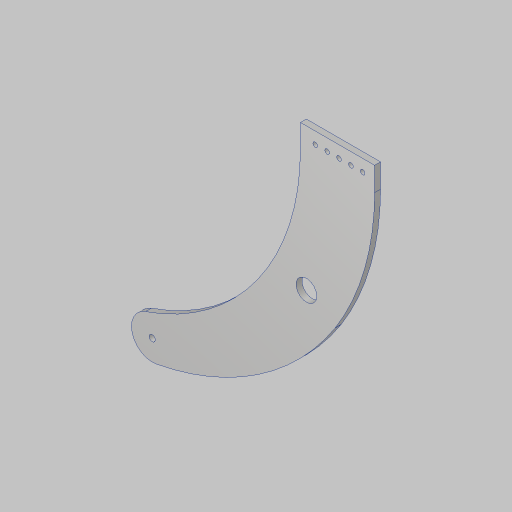
# Autodesk Inventor part: CL7-008
Saved by Autodesk Inventor 2023.5 (Build 275446000, 446)
## iProperties
Created: 2025-03-17
Part Number: CL7-008
Material: Aluminum 6061
Document SubType Name: Modeling
Designer: slick
Density: 2.7 g/cm^3
Appearance: Aluminum - Flat
Author: slick
Autodesk Inventor part; units mm, degrees
ref_plane "YZ Plane" through (0, 0, 0) normal (1, 0, 0) x (0, 1, 0)
ref_plane "XZ Plane" through (0, 0, 0) normal (0, 1, 0) x (-1, 0, 0)
ref_plane "XY Plane" through (0, 0, 0) normal (0, 0, 1) x (1, 0, 0)
sketch "Sketch1" plane through (0, 0, 0) normal (0, 0, 1) x (1, 0, 0)
  line L0 (-149.225, 152.4) -> (73.025, 152.4) construction
  line L1 (73.025, 152.4) -> (73.025, 127) construction
  line L2 (73.025, 127) -> (-149.225, 127) construction
  line L3 (-149.225, 127) -> (-149.225, 152.4) construction
  circle A0 centre (-165.1, -127) radius 12.7 construction
  circle A1 centre (0, 0) radius 23.8125 construction
  circle A2 centre (0, 0) radius 11.1125
  circle A3 centre (0, 0) radius 36.5125 construction
  line L4 (73.025, 152.4) -> (73.025, 127)
  line L5 (73.025, 152.4) -> (-6.4223, 152.4)
  line L6 (-6.4223, 152.4) -> (-6.4223, 127)
  circle A4 centre (-165.1, -127) radius 22.225 construction
  arc A5 (-172.3658, -105.9962) -> (-6.4223, 127) centre (-252.9655, 127) ccw
  arc A6 (-160.9917, -148.842) -> (30.7123, -19.7463) centre (-214.9861, 138.2242) ccw
  arc A7 (-172.3658, -105.9962) -> (-160.9917, -148.842) centre (-165.1, -127) ccw
  arc A8 (30.9373, -19.3918) -> (73.025, 127) centre (-202.6133, 127) ccw
  arc A9 (30.7123, -19.7463) -> (30.9373, -19.3918) centre (0, 0) ccw
  point P0 (60.325, 139.7)
  point P1 (73.025, 139.7)
  point P2 (47.625, 139.7)
  point P3 (34.925, 139.7)
  point P4 (22.225, 139.7)
  point P5 (9.525, 139.7)
  point P6 (30.9373, -19.3918)
  dimension "d0" = 25.4
  dimension "d1" = 127
  dimension "d2" = 222.25
  dimension "d3" = 149.225
  dimension "d4" = 25.4
  dimension "d5" = 127
  dimension "d6" = 165.1
  dimension "d7" = 12.7
  dimension "d8" = 47.625
  dimension "d9" = 22.225
  dimension "d12" = 12.7
  dimension "d17" = 12.7
  dimension "d18" = 9.525
  dimension "d19" = 292.1
  constraints: 15 point on circle, 14 end point, 10 centre point, 7 tangent, 5 coincident, 2 horizontal, 2 parallel, 2 perpendicular, 2 point on line, 1 horizontal alignment, 1 midpoint, 1 vertical, 4 other
  measures "d0" distance of L2.end L0.start
  measures "d1" distance from line of point (0, 0) L2
  measures "d2" distance of L0.start L0.end
  measures "d3" distance from line of point (0, 0) L3
  measures "d4" diameter of A0
  measures "d5" vertical distance of A0.centre point (0, 0)
  measures "d6" horizontal distance of A0.centre point (0, 0)
  measures "d7" distance from line of L1 point (60.325, 139.7)
  measures "d8" diameter of A1
  measures "d9" diameter of A2
  measures "d12" distance of point (60.325, 139.7) point (47.625, 139.7)
  measures "d17" radial gap between concentric circles of A1 A3
  measures "d18" radial gap between concentric circles of A0 A4
  measures "d19" radius of A6
extrude "Extrusion1" add sketch "Sketch1" along normal blind 6.35
hole "Hole1" at (60.325, 139.7, 0) at (47.625, 139.7, 0) at (34.925, 139.7, 0) at (22.225, 139.7, 0) at (9.525, 139.7, 0) direction (0, 0, 1) diameter 5.1054 end through all clearance for "Flat Head Machine Screw (82)" size "#10" standard "Ansi Unified Screw Threads"
hole "Hole2" at (-165.1, -127, 0) direction (0, 0, 1) diameter 6.7564 end through all clearance for "Flat Head Machine Screw (82)" size "1/4" standard "Ansi Unified Screw Threads"
body "Solid1"
